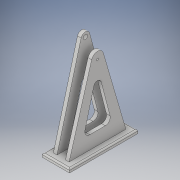
# Autodesk Inventor part: Stand
Saved by Autodesk Inventor 2017.1 (Build 211199000, 199)
## iProperties
Created: 2017-05-25
Part Number: Stand
Material: Generic
Document SubType Name: Modeling
Designer: 196918
Density: 1 g/cm^3
Appearance: Default
Author: 196918
Autodesk Inventor part; units mm, degrees
ref_plane "YZ Plane" through (0, 0, 0) normal (1, 0, 0) x (0, 1, 0)
sketch "Sketch1" plane through (0, 0, 0) normal (0, 1, 0) x (-1, 0, 0)
  line L0 (10.6955, 22.9336) -> (-69.3145, 22.9336)
  line L1 (-69.3145, 22.9336) -> (-69.3145, -176.9644)
  line L2 (-69.3145, -176.9644) -> (10.6955, -176.9644)
  line L3 (10.6955, -176.9644) -> (10.6955, 22.9336)
  point P0 (0, 0)
  dimension "d0" = 80.01
  dimension "d1" = 199.898
  constraints: 8 end point, 2 parallel, 1 horizontal, 1 perpendicular
  measures "d0" distance of L2.end L1.end
  measures "d1" distance of L1.end L0.end
extrude "Extrusion1" add sketch "Sketch1" along normal blind 10.668
fillet "Fillet1" radius 4.064 4 edges at (29.3095, 10.668, 22.9336) (69.3145, 10.668, -77.0154) (29.3095, 10.668, -176.9644) (-10.6955, 10.668, -77.0154)
ref_plane "Work Plane1" through (51.2805, 0, 22.9336) normal (1, 0, 0) x (0, 0, -1)
sketch "Sketch2" plane through (51.2805, 0, 22.9336) normal (1, 0, 0) x (0, 0, -1)
  line L0 (195.834, 10.668) -> (4.064, 10.668) construction
  line L1 (195.834, 10.668) -> (183.134, 10.668) construction
  arc A0 (4.064, 10.668) -> (0, 6.604) centre (4.064, 6.604) ccw construction
  line L2 (4.064, 10.668) -> (16.764, 10.668) construction
  line L3 (82.8788, 237.5782) -> (16.764, 10.668)
  line L4 (183.134, 10.668) -> (117.0192, 237.5782)
  line L5 (77.1008, 49.7952) -> (122.7972, 49.7952)
  line L6 (136.8055, 67.9313) -> (110.7624, 167.66)
  line L7 (89.1356, 167.66) -> (63.0925, 67.9313)
  arc A1 (117.0192, 237.5782) -> (82.8788, 237.5782) centre (99.949, 232.6044) ccw
  arc A2 (110.7624, 167.66) -> (89.1356, 167.66) centre (99.949, 164.8362) ccw
  arc A3 (63.0925, 67.9313) -> (77.1008, 49.7952) centre (77.1008, 64.2732) ccw
  arc A4 (122.7972, 49.7952) -> (136.8055, 67.9313) centre (122.7972, 64.2732) ccw
  line L8 (16.764, 10.668) -> (183.134, 10.668)
  point P0 (22.9336, 0)
  dimension "d6" = 12.7
  dimension "d7" = 12.7
  dimension "d9" = 17.78
  dimension "d10" = 11.176
  dimension "d11" = 14.478
  constraints: 16 end point, 8 point on circle, 8 tangent, 4 centre point, 2 point on line, 1 collinear, 1 equal radius, 1 horizontal
  measures "d6" distance of L0.start L1.end
  measures "d7" distance of L0.end L2.end
  measures "d9" radius of A1
  measures "d10" radius of A2
  measures "d11" radius of A3
extrude "Extrusion2" add sketch "Sketch2" against normal blind 10.668
sketch "Sketch3" plane through (51.2805, 0, 22.9336) normal (1, 0, 0) x (0, 0, -1)
  line L0 (16.764, 10.668) -> (183.134, 10.668) projected
  circle A0 centre (99.949, 229.8407) radius 3.048
  point P0 (22.9336, 0)
  dimension "d15" = 6.096
  constraints: 1 centre point
  measures "d15" diameter of A0
extrude "Extrusion3" cut sketch "Sketch3" against normal up to next
ref_plane "Work Plane2" through (5.0525, 0, -176.9644) normal (-1, 0, 0) x (0, 0, 1)
sketch "Sketch4" plane through (5.0525, 0, -176.9644) normal (-1, 0, 0) x (0, 0, 1)
  line L0 (16.764, 10.668) -> (183.134, 10.668) projected
  line L1 (117.0192, 237.5782) -> (183.134, 10.668) projected
  line L2 (16.764, 10.668) -> (183.134, 10.668)
  line L3 (16.764, 10.668) -> (87.4428, 272.4493)
  line L4 (112.4552, 272.4493) -> (183.134, 10.668)
  line L5 (16.764, 10.668) -> (183.134, 10.668)
  line L6 (77.1396, 43.0817) -> (122.7584, 43.0817)
  line L7 (136.7593, 61.2458) -> (110.7567, 160.0105)
  line L8 (89.1413, 160.0105) -> (63.1387, 61.2458)
  arc A0 (110.7567, 160.0105) -> (89.1413, 160.0105) centre (99.949, 157.1651) ccw
  arc A1 (63.1387, 61.2458) -> (77.1396, 43.0817) centre (77.1396, 57.5597) ccw
  arc A2 (122.7584, 43.0817) -> (136.7593, 61.2458) centre (122.7584, 57.5597) ccw
  line L9 (16.764, 10.668) -> (183.134, 10.668)
  arc A3 (112.4552, 272.4493) -> (87.4428, 272.4493) centre (99.949, 269.0728) ccw
  point P0 (176.9644, 0)
  point P1 (99.949, 318.77)
  point P2 (99.949, 201.0611)
  dimension "d21" = 11.176
  dimension "d22" = 14.478
  dimension "d25" = 12.954
  constraints: 16 end point, 8 point on circle, 8 tangent, 4 centre point, 4 point on line, 2 collinear, 2 horizontal, 1 equal radius
  measures "d21" radius of A0
  measures "d22" radius of A1
  measures "d25" radius of A3
extrude "Extrusion4" add sketch "Sketch4" against normal blind 10.668
sketch "Sketch5" plane through (5.0525, 0, -176.9644) normal (-1, 0, 0) x (0, 0, 1)
  arc A0 (112.4552, 272.4493) -> (87.4428, 272.4493) centre (99.949, 269.0728) ccw projected
  circle A1 centre (99.949, 269.0728) radius 6.477
  point P0 (176.9644, 0)
  dimension "d26" = 12.954
  constraints: 1 centre point, 1 coincident
  measures "d26" diameter of A1
extrude "Extrusion5" cut sketch "Sketch5" against normal up to next
body "Solid1"
